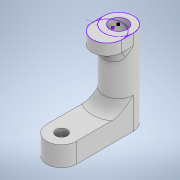
# Autodesk Inventor part: OBS-Mounting-A-003_LockingPin_v0.1.3
Saved by Autodesk Inventor 2021.1 (Build 251245010, 245A)
## iProperties
Created: 2021-03-10
Part Number: OBS-Mounting-A-003_LockingPin_v0.1.3
Material: Generisch
Document SubType Name: Modeling
Designer: hpcthobs
Density: 1 g/cm^3
Appearance: Vorgabe
Author: hpcthobs
Autodesk Inventor part; units mm, degrees
ref_plane "YZ Plane" through (0, 0, 0) normal (1, 0, 0) x (0, 1, 0)
ref_plane "XZ Plane" through (0, 0, 0) normal (0, 1, 0) x (-1, 0, 0)
ref_plane "XY Plane" through (0, 0, 0) normal (0, 0, 1) x (1, 0, 0)
sketch "Skizze1" plane through (-0.6517, 15, 4.517) normal (0, 1, 0) x (-1, 0, 0)
  circle A0 centre (-0.6517, -4.517) radius 1.5005
  circle A1 centre (-0.6517, -2.517) radius 2.6
  line L0 (-0.6517, -4.517) -> (-0.6517, -2.517) construction
  line L1 (-3.2517, -4.517) -> (-3.2517, -2.517)
  line L2 (1.9483, -2.517) -> (1.9483, -4.517)
  arc A2 (-3.2517, -4.517) -> (1.9483, -4.517) centre (-0.6517, -4.517) ccw
  arc A3 (1.9483, -2.517) -> (-3.2517, -2.517) centre (-0.6517, -2.517) ccw
  circle A4 centre (-0.6517, -4.517) radius 2.6
  point P0 (1.9483, -2.517)
  point P1 (-0.6517, -3.517)
  point P2 (1.9483, -2.517)
  point P3 (0.8434, -4.6441)
  point P4 (1.9483, -4.517)
  point P5 (-2.1468, -4.6441)
  constraints: 8 end point, 5 centre point, 4 point on circle, 4 tangent, 2 coincident, 1 concentric, 1 midpoint, 1 parallel, 1 vertical
extrude "Extrusion1" add sketch "Skizze1" against normal blind 2 contours A0 A1 A4 | A0 A1 A4 A2 | A4 L1 A1 | A1 A4 | A1 L2 A4
extrude "Extrusion2" add sketch "Skizze1" against normal blind 11.5 contours A0 A1 A4 | A0 A1 A4 A2
fillet "Rundung1" radius 2 1 edges at (0, 13, 2.6)
sketch "Skizze2" plane through (2.6, 0, 10) normal (0, -1, 0) x (1, 0, 0)
  line L0 (0, -8) -> (0, -10) projected
  circle A0 centre (-2.6, -10) radius 2.6
  circle A1 centre (-2.6, -10) radius 1.5005
  line L1 (-2.6, 0) -> (-2.6, -10) construction
  line L2 (-5.2, 0) -> (-5.2, -10)
  line L3 (0, -10) -> (0, 0)
  arc A2 (0, 0) -> (-5.2, 0) centre (-2.6, 0) ccw
  arc A3 (-5.2, -10) -> (0, -10) centre (-2.6, -10) ccw
  point P0 (-2.6, -5)
  constraints: 8 end point, 4 point on circle, 4 tangent, 3 centre point, 2 coincident, 1 midpoint, 1 parallel, 1 vertical, 3 other
extrude "Extrusion3" add sketch "Skizze2" against normal blind 3.5
fillet "Rundung2" radius 2 1 edges at (0, 3.5, 2.6)
sketch "Skizze3" plane through (2.6, 0, 10) normal (0, -1, 0) x (1, 0, 0)
  circle A0 centre (-2.6, 0) radius 1
  point P0 (-2.6, -10)
  dimension "d9" = 2
  constraints: 1 centre point
  measures "d9" diameter of A0
extrude "Extrusion4" cut sketch "Skizze3" against normal up to surface (3.5 mm away)
